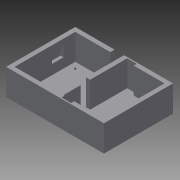
# Autodesk Inventor part: DelCo_2012_West_Structure
Saved by Autodesk Inventor 2014 (Build 180170000, 170)
## iProperties
Created: 2015-11-03
Part Number: DelCo_2012_West_Structure
Material: Generic
Document SubType Name: Modeling
Designer: jmw3
Density: 1 g/cm^3
Appearance: Default
Author: jmw3
Autodesk Inventor part; units mm, degrees
ref_plane "YZ Plane" through (0, 0, 0) normal (1, 0, 0) x (0, 1, 0)
ref_plane "XZ Plane" through (0, 0, 0) normal (0, 1, 0) x (-1, 0, 0)
ref_plane "XY Plane" through (0, 0, 0) normal (0, 0, 1) x (1, 0, 0)
sketch "Sketch1" plane through (0, 0, 0) normal (0, 1, 0) x (-1, 0, 0)
  line L0 (0, -4550) -> (0, 4550) projected
  line L1 (6440, 0) -> (-6440, 0) projected
  line L2 (0, -4550) -> (0, 4550) projected
  line L3 (-6440, 0) -> (6440, 0) projected
  line L4 (-1400, 2850) -> (-1400, 3250)
  line L5 (-500, 3250) -> (-500, 2850)
  line L6 (-4200, 2850) -> (-1400, 2850)
  line L7 (-4600, 3250) -> (-1400, 3250)
  line L8 (-500, 3250) -> (4600, 3250)
  line L9 (-1300, -3250) -> (-1300, -2850)
  line L10 (0, -3250) -> (-400, -3250)
  line L11 (-400, -3250) -> (-400, 350)
  line L12 (-400, 350) -> (0, 350)
  line L13 (0, 350) -> (0, -3250)
  line L14 (0, 3250) -> (-400, 3250)
  line L15 (-400, 2850) -> (-400, 1250)
  line L16 (-400, 1250) -> (0, 1250)
  line L17 (0, 1250) -> (0, 2850)
  line L18 (900, -3250) -> (900, -2850)
  line L19 (-500, 2850) -> (-400, 2850)
  line L20 (0, 2850) -> (4200, 2850)
  line L21 (-4200, -2850) -> (-4200, 750)
  line L22 (-4200, 1850) -> (-4200, 2850)
  line L23 (-4600, -3250) -> (-4600, 750)
  line L24 (-4600, 1850) -> (-4600, 3250)
  line L25 (4600, 3250) -> (4600, -650)
  line L26 (4600, -1750) -> (4600, -3250)
  line L27 (4200, 2850) -> (4200, -650)
  line L28 (4200, -1750) -> (4200, -2850)
  line L29 (4200, -2850) -> (900, -2850)
  line L30 (-1300, -2850) -> (-4200, -2850)
  line L31 (4600, -3250) -> (900, -3250)
  line L32 (-1300, -3250) -> (-4600, -3250)
  line L33 (-4600, 1850) -> (-4600, 750)
  line L34 (-4200, 1850) -> (-4200, 750)
  line L35 (4200, -1750) -> (4200, -650)
  line L36 (4600, -650) -> (4600, -1750)
  point P0 (0, 0)
  dimension "d5" = 900
  dimension "d11" = 900
  dimension "d12" = 400
  dimension "d14" = 900
  dimension "d19" = 6500
  dimension "d20" = 5700
  dimension "d21" = 1600
  dimension "d22" = 3600
  dimension "d23" = 9200
  dimension "d24" = 8400
  dimension "d25" = 2800
  constraints: 66 end point, 25 parallel, 20 perpendicular, 12 collinear, 6 horizontal, 5 point on line, 4 other
  measures "d5" distance between parallel lines of L5 L4
  measures "d11" distance between parallel lines of L9 L11
  measures "d12" distance between parallel lines of L11 L13
  measures "d14" distance between parallel lines of L2 L18
  measures "d19" distance between parallel lines of L8 L31
  measures "d20" distance between parallel lines of L20 L29
  measures "d21" distance between parallel lines of L20 L16
  measures "d22" distance between parallel lines of L10 L12
  measures "d23" distance between parallel lines of L23 L26
  measures "d24" distance between parallel lines of L21 L28
  measures "d25" distance between parallel lines of L22 L4
extrude "Extrusion1" add sketch "Sketch1" along normal blind 2438.4 contours L0 L1 L11 L12 | L16 L15 L19 L5 L8 L0 | L0 L10 L11 L1 | L0 L8 L25 L1 L27 L20 | L1 L25 L36 L26 L31 L18 L29 L28 L35 L27 | L21 L30 L9 L32 L23 L1 | L1 L23 L33 L24 L7 L4 L6 L22 L34 L21
sketch "Sketch2" plane through (0, 0, 0) normal (0, -1, 0) x (1, 0, 0)
  line L0 (-4600, -3250) -> (-4600, 3250) projected
  line L1 (-900, -3250) -> (-4600, -3250) projected
  line L2 (-900, -2850) -> (-900, -3250) projected
  line L3 (-4200, -2850) -> (-900, -2850) projected
  line L4 (-4200, 2850) -> (-4200, -2850) projected
  line L5 (0, 2850) -> (-4200, 2850) projected
  line L6 (0, 1250) -> (0, 2850) projected
  line L7 (400, 1250) -> (0, 1250) projected
  line L8 (400, 2850) -> (400, 1250) projected
  line L9 (500, 2850) -> (400, 2850) projected
  line L10 (500, 3250) -> (500, 2850) projected
  line L11 (-4600, 3250) -> (500, 3250) projected
  line L12 (-4600, 3250) -> (4600, 3250)
  line L13 (4600, 3250) -> (4600, -3250)
  line L14 (4600, -3250) -> (-4600, -3250)
  line L15 (-4600, -3250) -> (-4600, 3250)
  point P0 (0, 0)
  constraints: 8 end point, 2 parallel, 1 horizontal, 1 perpendicular
extrude "Extrusion2" add sketch "Sketch2" along normal blind 25.4
sketch "Sketch3" plane through (0, 2438.4, 0) normal (0, 1, 0) x (1, 0, 0)
  line L0 (1400, -3250) -> (4600, -3250) projected
  line L1 (4600, -3250) -> (4600, 3250) projected
  line L2 (4600, 3250) -> (1300, 3250) projected
  line L3 (1300, 3250) -> (1300, 2850) projected
  line L4 (1300, 2850) -> (4200, 2850) projected
  line L5 (4200, 2850) -> (4200, -2850) projected
  line L6 (4200, -2850) -> (1400, -2850) projected
  line L7 (1400, -2850) -> (1400, -3250) projected
  line L8 (400, -350) -> (400, 3250) projected
  line L9 (400, 3250) -> (0, 3250) projected
  line L10 (0, 3250) -> (0, -350) projected
  line L11 (0, -350) -> (400, -350) projected
  line L12 (500, -3250) -> (1400, -3250)
  line L13 (1400, -3250) -> (1400, -3135.7)
  line L14 (1400, -3135.7) -> (500, -3135.7)
  line L15 (500, -3135.7) -> (500, -3250)
  line L16 (400, 3250) -> (1300, 3250)
  line L17 (1300, 3250) -> (1300, 3135.7)
  line L18 (1300, 3135.7) -> (400, 3135.7)
  line L19 (400, 3135.7) -> (400, 3250)
  point P0 (0, 0)
  dimension "d31" = 114.3
  dimension "d33" = 114.3
  constraints: 16 end point, 4 parallel, 2 horizontal, 2 perpendicular, 2 point on line
  measures "d31" distance between parallel lines of L12 L14
  measures "d33" distance between parallel lines of L16 L18
extrude "Extrusion3" add sketch "Sketch3" against normal up to surface (2438.4 mm away) contours L12 L15 L14 L7 | L3 L18 L8 L16
sketch "Sketch4" plane through (-4200, 2438.4, 2850) normal (1, 0, 0) x (0, 0, -1)
  line L0 (0, -2438.4) -> (5700, -2438.4) projected
  line L1 (5700, -2438.4) -> (5700, 0) projected
  line L2 (3500, -524) -> (4600, -524)
  line L3 (4600, -524) -> (4600, -1524)
  line L4 (4600, -1524) -> (3500, -1524)
  line L5 (3500, -1524) -> (3500, -524)
  point P0 (2850, -2438.4)
  dimension "d36" = 1100
  dimension "d37" = 1100
  dimension "d38" = 914.4
  dimension "d39" = 1000
  constraints: 8 end point, 2 parallel, 1 horizontal, 1 perpendicular
  measures "d36" distance between parallel lines of L3 L5
  measures "d37" distance between parallel lines of L1 L3
  measures "d38" distance between parallel lines of L0 L4
  measures "d39" distance between parallel lines of L4 L2
extrude "Extrusion4" cut sketch "Sketch4" against normal blind 285.75
sketch "Sketch5" plane through (4200, 2438.4, -2850) normal (-1, 0, 0) x (0, 0, 1)
  line L0 (5700, -2438.4) -> (0, -2438.4) projected
  line L1 (5700, -2438.4) -> (5700, 0) projected
  line L2 (3600, -524) -> (4700, -524)
  line L3 (4700, -524) -> (4700, -1524)
  line L4 (4700, -1524) -> (3600, -1524)
  line L5 (3600, -1524) -> (3600, -524)
  point P0 (2850, -2438.4)
  dimension "d42" = 1000
  dimension "d43" = 1100
  dimension "d44" = 1000
  dimension "d45" = 914.4
  constraints: 8 end point, 2 parallel, 1 horizontal, 1 perpendicular
  measures "d42" distance between parallel lines of L1 L3
  measures "d43" distance between parallel lines of L3 L5
  measures "d44" distance between parallel lines of L4 L2
  measures "d45" distance between parallel lines of L0 L4
extrude "Extrusion5" cut sketch "Sketch5" against normal blind 285.75
sketch "Sketch7" plane through (0, 0, 0) normal (0, 1, 0) x (1, 0, 0)
  line L0 (1400, -2850) -> (4200, -2850) projected
  line L1 (4200, -2850) -> (4200, 2850) projected
  line L2 (2900, 50) -> (3900, 50)
  line L3 (3900, 50) -> (3900, -1150)
  line L4 (3900, -1150) -> (2900, -1150)
  line L5 (2900, -1150) -> (2900, 50)
  line L6 (2900, -1350) -> (3900, -1350)
  line L7 (3900, -1350) -> (3900, -2550)
  line L8 (3900, -2550) -> (2900, -2550)
  line L9 (2900, -2550) -> (2900, -1350)
  point P0 (0, 0)
  dimension "d79" = 300
  dimension "d80" = 200
  dimension "d81" = 300
  dimension "d82" = 1200
  dimension "d83" = 1000
  dimension "d84" = 1200
  constraints: 16 end point, 4 parallel, 2 collinear, 2 horizontal, 2 perpendicular
  measures "d79" distance between parallel lines of L1 L3
  measures "d80" distance between parallel lines of L6 L4
  measures "d81" distance between parallel lines of L0 L8
  measures "d82" distance between parallel lines of L2 L4
  measures "d83" distance between parallel lines of L3 L5
  measures "d84" distance between parallel lines of L8 L6
extrude "Pallets" add sketch "Sketch7" along normal blind 152.4
sketch "Sketch6" plane through (0, 0, 0) normal (0, 1, 0) x (1, 0, 0)
  line L0 (400, -350) -> (400, 3135.7) projected
  line L1 (0, -350) -> (400, -350) projected
  line L2 (-900, 3250) -> (0, 3250) projected
  line L3 (-4200, 2850) -> (-900, 2850) projected
  line L4 (-4200, -2850) -> (-4200, 2850) projected
  line L5 (0, -2850) -> (-4200, -2850) projected
  line L6 (0, -1250) -> (0, -2850) projected
  circle A0 centre (700, -850) radius 76.2
  circle A1 centre (-3600, -2250) radius 76.2
  circle A2 centre (-3600, 2250) radius 76.2
  circle A3 centre (-600, -2250) radius 76.2
  line L7 (-2176.2, -126.2) -> (-2023.8, -126.2)
  line L8 (-2023.8, -126.2) -> (-2023.8, 26.2)
  line L9 (-2023.8, 26.2) -> (-2176.2, 26.2)
  line L10 (-2176.2, 26.2) -> (-2176.2, -126.2)
  line L11 (-2176.2, -126.2) -> (-2023.8, 26.2) construction
  line L12 (-2023.8, -126.2) -> (-2176.2, 26.2) construction
  line L13 (-526.2, 3173.8) -> (-373.8, 3173.8)
  line L14 (-526.2, 3326.2) -> (-526.2, 3173.8)
  line L15 (-526.2, 3173.8) -> (-373.8, 3326.2) construction
  line L16 (-373.8, 3173.8) -> (-526.2, 3326.2) construction
  line L17 (-526.2, 3326.2) -> (-373.8, 3173.8)
  point P0 (0, 0)
  point P1 (-2100, -50)
  point P2 (-450, 3250)
  dimension "d55" = 152.4
  dimension "d56" = 300
  dimension "d57" = 500
  dimension "d58" = 152.4
  dimension "d59" = 152.4
  dimension "d60" = 152.4
  dimension "d61" = 600
  dimension "d62" = 600
  dimension "d63" = 600
  dimension "d64" = 600
  dimension "d65" = 600
  dimension "d66" = 600
  dimension "d69" = 2800
  dimension "d70" = 2100
  dimension "d71" = 152.4
  dimension "d72" = 152.4
  dimension "d75" = 152.4
  dimension "d76" = 152.4
  constraints: 22 end point, 5 midpoint, 4 centre point, 3 equal length, 2 horizontal, 1 perpendicular
  measures "d55" diameter of A0
  measures "d56" distance from line of L0 A0.centre
  measures "d57" distance from line of L1 A0.centre
  measures "d58" diameter of A1
  measures "d59" diameter of A2
  measures "d60" diameter of A3
  measures "d61" distance from line of L5 A3.centre
  measures "d62" distance from line of L6 A3.centre
  measures "d63" distance from line of L4 A1.centre
  measures "d64" distance from line of L5 A1.centre
  measures "d65" distance from line of L4 A2.centre
  measures "d66" distance from line of L3 A2.centre
  measures "d69" distance from line of L5 point (-2100, -50)
  measures "d70" distance from line of L4 point (-2100, -50)
  measures "d71" distance of L9.end L8.end
  measures "d72" distance between parallel lines of L7 L9
  measures "d75" distance of L14.start L13.start
  measures "d76" distance of L13.start L13.end
extrude "Instrumentation" add sketch "Sketch6" along normal blind 152.4
body "Solid1"
